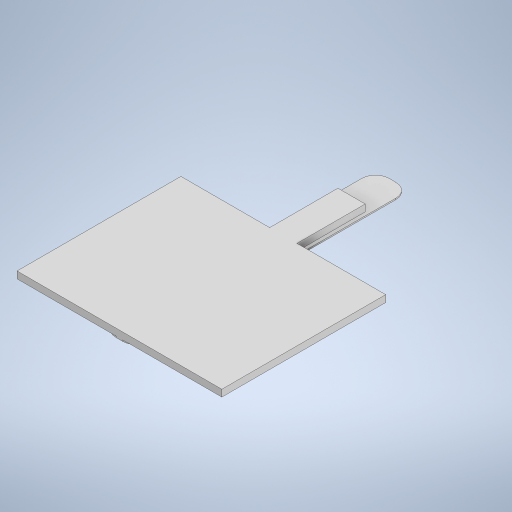
# Autodesk Inventor part: base
Saved by Autodesk Inventor 2023 (Build 270158000, 158)
## iProperties
Created: 2023-01-20
Part Number: base
Material: Generic
Document SubType Name: Modeling
Designer: kavya
Density: 1 g/cm^3
Appearance: Default
Author: kavya
Autodesk Inventor part; units mm, degrees
ref_plane "YZ Plane" through (0, 0, 0) normal (1, 0, 0) x (0, 1, 0)
ref_plane "XZ Plane" through (0, 0, 0) normal (0, 1, 0) x (-1, 0, 0)
ref_plane "XY Plane" through (0, 0, 0) normal (0, 0, 1) x (1, 0, 0)
sketch "Sketch1" plane through (0, 0, 0) normal (0, 1, 0) x (-1, 0, 0)
  line L0 (0, 0) -> (-150, 0)
  line L1 (-150, 0) -> (-150, -120)
  line L2 (0, -120) -> (0, 0)
  line L3 (-65, -120) -> (-85, -120)
  line L4 (-85, -120) -> (-85, -170)
  line L5 (-85, -170) -> (-65, -170)
  line L6 (-65, -170) -> (-65, -120)
  line L7 (-150, -120) -> (-85, -120)
  line L8 (-65, -120) -> (0, -120)
  dimension "d0" = 150
  dimension "d1" = 120
  dimension "d2" = 20
  dimension "d3" = 50
  constraints: 18 end point, 5 parallel, 2 horizontal, 2 perpendicular
  measures "d0" distance of L2.start L1.end
  measures "d1" distance of L1.end L0.end
  measures "d2" distance of L5.end L4.end
  measures "d3" distance of L4.end L3.end
extrude "Extrusion1" add sketch "Sketch1" along normal blind 5
sketch "Sketch2" plane through (0, 0, 0) normal (0, -1, 0) x (1, 0, 0)
  line L0 (0, 0) -> (150, 0) projected
  line L1 (77.5, 0) -> (72.5, 0)
  line L2 (62.5, -10) -> (62.5, -190)
  line L3 (72.5, -200) -> (77.5, -200)
  line L4 (87.5, -190) -> (87.5, -10)
  arc A0 (62.5, -190) -> (72.5, -200) centre (72.5, -190) ccw
  arc A1 (77.5, -200) -> (87.5, -190) centre (77.5, -190) ccw
  arc A2 (72.5, 0) -> (62.5, -10) centre (72.5, -10) ccw
  arc A3 (87.5, -10) -> (77.5, 0) centre (77.5, -10) ccw
  point P0 (87.5, 0)
  point P1 (62.5, -200)
  point P2 (62.5, 0)
  point P3 (87.5, -200)
  dimension "d6" = 25
  dimension "d7" = 200
  dimension "d8" = 10
  constraints: 9 point on line, 8 end point, 8 point on circle, 8 tangent, 4 centre point, 3 equal radius, 2 parallel, 1 horizontal, 1 perpendicular
  measures "d6" distance of point (87.5, -200) point (62.5, -200)
  measures "d7" distance of point (62.5, -200) point (62.5, 0)
  measures "d8" radius of A0
extrude "Extrusion2" add sketch "Sketch2" along normal blind 1
body "Solid1"
